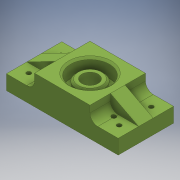
# Autodesk Inventor part: sujetador guia ejercedor presion
Saved by Autodesk Inventor 2018 (Build 220112000, 112)
## iProperties
Created: 2019-05-18
Part Number: sujetador guia ejercedor presion
Material: Generic
Document SubType Name: Modeling
Designer: JLVega003
Density: 1 g/cm^3
Appearance: Olive Green
Author: JLVega003
Autodesk Inventor part; units mm, degrees
ref_plane "YZ Plane" through (0, 0, 0) normal (1, 0, 0) x (0, 1, 0)
ref_plane "XZ Plane" through (0, 0, 0) normal (0, 1, 0) x (-1, 0, 0)
ref_plane "XY Plane" through (0, 0, 0) normal (0, 0, 1) x (1, 0, 0)
sketch "Sketch1" plane through (0, 0, 0) normal (0, 0, 1) x (1, 0, 0)
  line L0 (57.5, -28.5) -> (-57.5, -28.5)
  line L1 (-57.5, -28.5) -> (-57.5, 28.5)
  line L2 (-57.5, 28.5) -> (57.5, 28.5)
  line L3 (57.5, 28.5) -> (57.5, -28.5)
  line L4 (57.5, -28.5) -> (-57.5, 28.5) construction
  line L5 (-57.5, -28.5) -> (57.5, 28.5) construction
  line L6 (46.5, -16.5) -> (-46.5, -16.5) construction
  line L7 (-46.5, -16.5) -> (-46.5, 16.5) construction
  line L8 (-46.5, 16.5) -> (46.5, 16.5) construction
  line L9 (46.5, 16.5) -> (46.5, -16.5) construction
  line L10 (46.5, -16.5) -> (-46.5, 16.5) construction
  line L11 (-46.5, -16.5) -> (46.5, 16.5) construction
  line L12 (36, -11.5) -> (-36, -11.5) construction
  line L13 (-36, -11.5) -> (-36, 11.5) construction
  line L14 (-36, 11.5) -> (36, 11.5) construction
  line L15 (36, 11.5) -> (36, -11.5) construction
  line L16 (36, -11.5) -> (-36, 11.5) construction
  line L17 (-36, -11.5) -> (36, 11.5) construction
  circle A0 centre (-46.5, 16.5) radius 2.25
  circle A1 centre (-36, 11.5) radius 2.25
  circle A2 centre (-46.5, -16.5) radius 2.25
  circle A3 centre (-36, -11.5) radius 2.25
  circle A4 centre (46.5, -16.5) radius 2.25
  circle A5 centre (36, -11.5) radius 2.25
  circle A6 centre (36, 11.5) radius 2.25
  circle A7 centre (46.5, 16.5) radius 2.25
  point P0 (0, 0)
  dimension "d0" = 115
  dimension "d1" = 57
  dimension "d2" = 93
  dimension "d3" = 33
  dimension "d4" = 72
  dimension "d5" = 23
  dimension "d6" = 4.5
  constraints: 36 end point, 8 centre point, 8 coincident, 7 equal radius, 6 midpoint, 6 parallel, 3 horizontal, 3 perpendicular
  measures "d0" distance of L1.end L2.end
  measures "d1" distance of L0.end L1.end
  measures "d2" distance of L7.end L8.end
  measures "d3" distance of L6.end L7.end
  measures "d4" distance of L13.end L14.end
  measures "d5" distance of L12.end L13.end
  measures "d6" diameter of A0
extrude "Extrusion1" add sketch "Sketch1" along normal blind 15
sketch "Sketch2" plane through (0, 0, 0) normal (0, 0, -1) x (-1, 0, 0)
  circle A0 centre (-46.5, 16.5) radius 2.25 projected
  circle A1 centre (-36, 11.5) radius 2.25 projected
  circle A2 centre (-36, -11.5) radius 2.25 projected
  circle A3 centre (-46.5, -16.5) radius 2.25 projected
  circle A4 centre (36, -11.5) radius 2.25 projected
  circle A5 centre (46.5, -16.5) radius 2.25 projected
  circle A6 centre (36, 11.5) radius 2.25 projected
  circle A7 centre (46.5, 16.5) radius 2.25 projected
  line L0 (-57.5, -28.5) -> (57.5, -28.5) projected
  line L1 (57.5, -28.5) -> (57.5, 28.5) projected
  line L2 (57.5, 28.5) -> (-57.5, 28.5) projected
  line L3 (-57.5, 28.5) -> (-57.5, -28.5) projected
  circle A8 centre (-46.5, 16.5) radius 2.25 projected
  circle A9 centre (-46.5, 16.5) radius 6
  circle A10 centre (-46.5, -16.5) radius 2.25 projected
  circle A11 centre (-46.5, -16.5) radius 6
  circle A12 centre (46.5, -16.5) radius 6
  circle A13 centre (46.5, 16.5) radius 6
  point P0 (0, 0)
  dimension "d9" = 12
  constraints: 4 centre point, 4 coincident, 3 equal radius
  measures "d9" diameter of A9
extrude "Extrusion2" cut sketch "Sketch2" against normal blind 7 contours A9 | A11 | A12 | A13
sketch "Sketch3" plane through (0, 0, 15) normal (0, 0, 1) x (1, 0, 0)
  line L0 (-57.5, -28.5) -> (57.5, -28.5) projected
  line L1 (28.5, 28.5) -> (-28.5, 28.5)
  line L2 (-28.5, 28.5) -> (-28.5, -28.5)
  line L3 (-28.5, -28.5) -> (28.5, -28.5)
  line L4 (28.5, -28.5) -> (28.5, 28.5)
  line L5 (28.5, 28.5) -> (-28.5, -28.5) construction
  line L6 (-28.5, 28.5) -> (28.5, -28.5) construction
  point P0 (0, 0)
  dimension "d12" = 57
  constraints: 12 end point, 2 midpoint, 2 parallel, 1 horizontal, 1 perpendicular, 1 point on line
  measures "d12" distance of L3.end L2.end
extrude "Extrusion3" add sketch "Sketch3" along normal blind 15
fillet "Fillet1" radius 8 2 edges at (-28.5, 0, 15) (28.5, 0, 15)
sketch "Sketch4" plane through (0, 0, 0) normal (0, 1, 0) x (-1, 0, 0)
  line L0 (-57.5, 0) -> (57.5, 0) projected
  line L1 (-57.5, 0) -> (-57.5, 15) projected
  line L2 (-36.5, 15) -> (-57.5, 15) projected
  arc A0 (-36.5, 15) -> (-28.5, 23) centre (-36.5, 23) ccw projected
  line L3 (-28.5, 23) -> (-28.5, 30) projected
  line L4 (28.5, 30) -> (-28.5, 30) projected
  line L5 (28.5, 23) -> (28.5, 30) projected
  arc A1 (28.5, 23) -> (36.5, 15) centre (36.5, 23) ccw projected
  line L6 (57.5, 15) -> (36.5, 15) projected
  line L7 (57.5, 0) -> (57.5, 15) projected
  line L8 (28.5, 30) -> (57.5, 15)
  line L9 (-28.5, 23) -> (-28.5, 30) projected
  line L10 (-28.5, 30) -> (-57.5, 15)
  line L11 (-28.5, 30) -> (-28.5, 15)
  line L12 (-28.5, 15) -> (-57.5, 15)
  line L13 (28.5, 23) -> (28.5, 30) projected
  line L14 (28.5, 30) -> (28.5, 15)
  line L15 (28.5, 15) -> (57.5, 15)
  point P0 (0, 0)
  constraints: 12 end point, 2 perpendicular, 1 collinear, 1 point on line, 1 vertical
extrude "Extrusion4" add sketch "Sketch4" along normal mid plane 15 contours L10 L3 A0 L2 | L6 A1 L5 L8
sketch "Sketch5" plane through (0, 0, 0) normal (0, 1, 0) x (-1, 0, 0)
  line L0 (0, -6) -> (0, 36) projected
  line L1 (0, 0) -> (0, 30)
  line L2 (28.5, 30) -> (-28.5, 30) projected
  line L3 (0, 30) -> (20, 30)
  line L4 (20, 30) -> (20, 15)
  line L5 (20, 15) -> (14, 15)
  line L6 (14, 15) -> (14, 25)
  line L7 (14, 25) -> (8.4, 25)
  line L8 (8.4, 25) -> (8.4, 0)
  line L9 (8.4, 0) -> (0, 0)
  dimension "d18" = 40
  dimension "d19" = 28
  dimension "d20" = 16.8
  dimension "d21" = 5
  dimension "d22" = 15
  constraints: 16 end point, 5 perpendicular, 1 midpoint, 1 point on line, 1 vertical
  measures "d18" diameter of L4 L0
  measures "d19" diameter of L6 L0
  measures "d20" diameter of L8 L0
  measures "d21" distance between parallel lines of L7 L2
  measures "d22" distance between parallel lines of L5 L2
revolve "Revolution1" cut sketch "Sketch5" angle 360 about axis through (0, 0, -10) along (0, 0, 1)
chamfer "Chamfer1" distance 2 angle 45 3 edges at (20, 0, 30) (14, 0, 25) (8.4, 0, 0)
body "Solid1"
